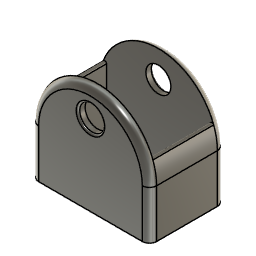
Big Safety Pin Lock v2 (Autodesk Fusion 360 design; units mm, degrees)
Autodesk Fusion 360 part; units mm, degrees
sketch "Sketch1" plane through (0, 0, 0) normal (0, 0, 1) x (1, 0, 0)
  line L0 (0, 0) -> (14.5, 0)
  line L1 (14.5, 0) -> (14.5, 8.5)
  line L2 (14.5, 8.5) -> (0, 8.5)
  line L3 (0, 8.5) -> (0, 0)
  dimension "d1" = 14.5
  dimension "d2" = 8.5
  constraint horizontal L0
  constraint vertical L1
  constraint horizontal L2
  constraint vertical L3
  constraint coincident L0.start L3.end
  measures "d1" distance of L0.start L0.end
  measures "d2" distance of L0.start L2.end
extrude "Extrude1" add sketch "Sketch1" along normal blind 15 makes body 1
copy_body "Body->Comp1" bodies 1 removing the originals makes body 2 in component "Template"
sketch "Sketch1 (2)" plane through (0, 0, 0) normal (0, 0, 1) x (1, 0, 0) in component "LockCollar"
  line L0 (14.5, 8.5) -> (0, 8.5)
  line L1 (0, 8.5) -> (0, 0)
  line L2 (0, 0) -> (14.5, 0)
  line L3 (14.5, 0) -> (14.5, 8.5)
  line L4 (0, 8.5) -> (14.5, 8.5)
  line L5 (14.5, 8.5) -> (14.5, 0)
  line L6 (14.5, 0) -> (0, 0)
  line L7 (0, 0) -> (0, 8.5)
  line L8 (0, 8.5) -> (14.5, 0) construction
  line L9 (15.5, -1) -> (-1, -1)
  line L10 (-1, -1) -> (-1, 9.5)
  line L11 (-1, 9.5) -> (15.5, 9.5)
  line L12 (15.5, 9.5) -> (15.5, -1)
  line L13 (15.5, -1) -> (-1, 9.5) construction
  line L14 (-1, -1) -> (15.5, 9.5) construction
  point P0 (7.25, 4.25)
  dimension "d5" = 16.5
  dimension "d6" = 10.5
  constraint horizontal L4
  constraint vertical L5
  constraint horizontal L6
  constraint vertical L7
  constraint coincident L2.end L3.start
  constraint coincident L0.end L1.start
  constraint horizontal L9
  constraint perpendicular L9 L10
  constraint parallel L9 L11
  constraint parallel L10 L12
  constraint coincident L13 P0
  constraint coincident L14 P0
  constraint midpoint L8 P0
  measures "d5" distance of L10.end L11.end
  measures "d6" distance of L9.end L10.end
extrude "Extrude1'" add sketch "Sketch1 (2)" along normal blind 15 separate body makes body 3 in component "LockCollar"
sketch "Sketch2" plane through (0, -1, 0) normal (0, -1, 0) x (1, 0, 0) in component "LockCollar"
  line L0 (-1, 0) -> (15.5, 0)
  line L1 (15.5, 0) -> (15.5, 15)
  line L2 (15.5, 15) -> (-1, 15)
  line L3 (-1, 15) -> (-1, 0)
  line L4 (7.25, 15) -> (7.25, 11.75) construction
  circle A0 centre (7.25, 11.75) radius 1.25
  dimension "d9" = 3.25
  dimension "d10" = 2.5
  constraint midpoint L2 L4.start
  constraint perpendicular L2 L4
  constraint coincident L4.end A0.centre
  measures "d9" distance of L4.start L4.end
  measures "d10" diameter of A0
extrude "Extrude1''" cut sketch "Sketch2" against normal blind 10.5 contours A0 bodies 2 in component "Template"
extrude "Extrude2" cut sketch "Sketch2" against normal blind 10.5 contours A0 bodies 3 in component "LockCollar"
fillet "Fillet1" radius 8.25 2 edges at (15.5, 4.25, 15) (-1, 4.25, 15) on bodies 3 in component "LockCollar"
fillet "Fillet2" radius 1 6 edges at (-1, -1, 3.375) (7.25, -1, 15) (15.5, -1, 3.375) (-1, 9.5, 3.375) (7.25, 9.5, 15) (15.5, 9.5, 3.375) on bodies 3 in component "LockCollar"
fillet "Fillet3" radius 0.25 1 edges at (0, 4.25, 10.687) on bodies 3 in component "LockCollar"
fillet "Fillet4" radius 0.25 1 edges at (14.5, 4.25, 10.687) on bodies 3 in component "LockCollar"
fillet "Fillet5" radius 0.25 1 edges at (7.25, 0, 0) on bodies 3 in component "LockCollar"
fillet "Fillet6" radius 0.25 1 edges at (7.25, 8.5, 0) on bodies 3 in component "LockCollar"
fillet "Fillet7" radius 0.25 1 edges at (14.5, 4.25, 0) on bodies 3 in component "LockCollar"
fillet "Fillet8" radius 0.25 1 edges at (0, 4.25, 0) on bodies 3 in component "LockCollar"
copy_body "CopyPasteBodies1" bodies 3 makes body 4
move_body "Move1" bodies 4 to x (1, 0, 0) y (0, 1, 0) z (0, 0, 1) at (0, 0, 0)
copy_body "Body->Comp2" bodies 4 removing the originals makes body 5 in component "LockCollarPadlock"
move_body "Move1'" bodies 5 to x (1, 0, 0) y (0, 1, 0) z (0, 0, 1) at (25, 0, 0) in component "LockCollarPadlock"
sketch "Sketch2 (2)" plane through (0, -1, 0) normal (0, -1, 0) x (1, 0, 0)
  circle A0 centre (32.25, 11.75) radius 1.25
  line L0 (39.5, 0) -> (39.5, 6.75)
  arc A1 (39.5, 6.75) -> (25, 6.75) centre (32.25, 6.75) ccw
  line L1 (25, 6.75) -> (25, 0)
  line L2 (25, 0) -> (39.5, 0)
  line L3 (32.25, 13) -> (32.25, 10.5) construction
  line L4 (32.25, 13) -> (32.25, 11.25) construction
  circle A2 centre (32.25, 11.25) radius 1.75
  dimension "d31" = 1.75
  dimension "d32" = 3.5
  constraint coincident A0 L3.start
  constraint parallel L3 L4
  constraint coincident A0 L3.end
  constraint coincident L4.end A2.centre
  measures "d31" distance of L3.start L4.end
  measures "d32" diameter of A2
extrude "Extrude1'''" cut sketch "Sketch2 (2)" against normal blind 10.5 contours A2 bodies 5 in component "LockCollarPadlock"
fillet "Fillet1'" radius 0.25 1 edges at (30.6184, -1, 11.8828) on bodies 5 in component "LockCollarPadlock"
fillet "Fillet2'" radius 0.25 1 edges at (30.6184, 9.5, 10.6172) on bodies 5 in component "LockCollarPadlock"
component "Template" placed x (1, 0, 0) y (0, 1, 0) z (0, 0, 1) at (0, 0, 0)
component "LockCollar" placed x (1, 0, 0) y (0, 1, 0) z (0, 0, 1) at (0, 0, 0)
component "LockCollarPadlock" placed x (1, 0, 0) y (0, 1, 0) z (0, 0, 1) at (0, 0, 0)
hidden bodies 3
equation "d9 = 2 mm + 1.25 mm"
equation "d31 = ( 3.5 / 2 ) * 1 mm"
